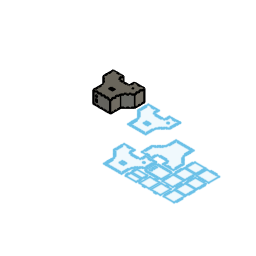
JD_BopIt_Enclosure (Autodesk Fusion 360 design; units mm, degrees)
Autodesk Fusion 360 part; units mm, degrees
(part 1 of 2)
sketch "Base" plane through (0, 0, 0) normal (0, 0, 1) x (1, 0, 0)
  line L0 (6.35, 14.5143) -> (6.35, 27.2143)
  line L1 (6.35, 27.2143) -> (0, 27.2143)
  line L2 (0, 39.9143) -> (6.35, 39.9143)
  line L3 (6.35, 39.9143) -> (6.35, 52.6143)
  line L4 (6.35, 52.6143) -> (0.1301, 52.6143)
  line L5 (0.1661, 65.1641) -> (0.1301, 52.6143)
  line L6 (0, 39.9143) -> (0, 27.2143)
  line L7 (6.35, 14.5143) -> (6.35, 27.2143)
  line L8 (6.35, 27.2143) -> (0, 27.2143)
  line L9 (31.7482, 0) -> (31.7482, 6.35)
  line L10 (31.7482, 6.35) -> (19.0482, 6.35)
  line L11 (19.0482, 6.35) -> (19.0482, 0)
  line L12 (57.1482, 6.35) -> (44.4482, 6.35)
  line L13 (44.4482, 6.35) -> (44.4482, 0)
  line L14 (57.1482, 0) -> (57.1482, 6.35)
  line L15 (82.5482, 6.35) -> (69.8482, 6.35)
  line L16 (69.8482, 6.35) -> (69.8482, 0)
  line L17 (82.5482, 0) -> (82.5482, 6.35)
  line L18 (107.9482, 6.35) -> (95.2482, 6.35)
  line L19 (95.2482, 6.35) -> (95.2482, 0)
  line L20 (107.9482, 0) -> (107.9482, 6.35)
  line L21 (31.7482, 0) -> (44.4482, 0)
  line L22 (57.1482, 0) -> (69.8482, 0)
  line L23 (82.5482, 0) -> (95.2482, 0)
  line L24 (107.9482, 0) -> (112.4857, 0)
  line L25 (6.35, 14.5143) -> (6.35, 27.2143)
  line L26 (6.35, 27.2143) -> (0, 27.2143)
  line L27 (0, 39.9143) -> (6.35, 39.9143)
  line L28 (6.35, 39.9143) -> (6.35, 52.6143)
  line L29 (6.35, 52.6143) -> (0, 52.6143)
  line L30 (6.35, 14.5143) -> (6.35, 27.2143)
  line L31 (6.35, 27.2143) -> (0, 27.2143)
  line L32 (0, 39.9143) -> (6.35, 39.9143)
  line L33 (6.35, 39.9143) -> (6.35, 52.6143)
  line L34 (6.35, 52.6143) -> (0, 52.6143)
  line L35 (127, 14.5143) -> (120.65, 14.5143)
  line L36 (120.65, 14.5143) -> (120.65, 27.2143)
  line L37 (120.65, 27.2143) -> (127, 27.2143)
  line L38 (127, 39.9143) -> (120.65, 39.9143)
  line L39 (120.65, 39.9143) -> (120.65, 52.6143)
  line L40 (120.65, 52.6143) -> (127, 52.6143)
  line L41 (127, 27.2143) -> (127, 39.9143)
  line L42 (127, 52.6143) -> (127, 65.0564)
  line L43 (19.0482, 0) -> (14.5107, 0)
  line L44 (6.35, 14.5143) -> (-0.0036, 14.5143)
  line L45 (152.6542, 98.2256) -> (148.1641, 93.7355)
  line L46 (148.1641, 93.7355) -> (143.6703, 98.2293)
  line L47 (143.6703, 98.2293) -> (134.69, 89.249)
  line L48 (134.69, 89.249) -> (139.1839, 84.7552)
  line L49 (157.1443, 102.7158) -> (152.6579, 107.2022)
  line L50 (152.6579, 107.2022) -> (161.6381, 116.1825)
  line L51 (161.6381, 116.1825) -> (166.1246, 111.696)
  line L52 (132.3139, 77.8854) -> (139.1838, 84.7552)
  line L53 (148.1641, 93.7355) -> (157.1443, 102.7158)
  line L54 (166.1246, 111.696) -> (173.0018, 118.5733)
  line L55 (178.3158, 148.5091) -> (171.9658, 148.5091)
  line L56 (171.9658, 148.5091) -> (171.9658, 135.8091)
  line L57 (171.9658, 135.8091) -> (178.3158, 135.8091)
  line L58 (178.3158, 154.8591) -> (178.3158, 161.2091)
  line L59 (178.3158, 161.2091) -> (171.9658, 161.2091)
  line L60 (171.9658, 161.2091) -> (171.9658, 173.9091)
  line L61 (171.9658, 173.9091) -> (178.3158, 173.9091)
  line L62 (178.3158, 131.4022) -> (178.3158, 135.8091)
  line L63 (178.3158, 148.5091) -> (178.3158, 161.2091)
  line L64 (178.3158, 173.9091) -> (178.3158, 178.3158)
  line L65 (146.3553, 196.4586) -> (146.3553, 190.1086)
  line L66 (146.3553, 190.1086) -> (133.6553, 190.1086)
  line L67 (133.6553, 190.1086) -> (133.6553, 196.4586)
  line L68 (160.1729, 196.4586) -> (146.3553, 196.4586)
  line L69 (133.6553, 196.4586) -> (119.8377, 196.4586)
  line L70 (82.855, 160.1729) -> (82.855, 153.8229)
  line L71 (82.855, 153.8229) -> (70.155, 153.8229)
  line L72 (70.155, 153.8229) -> (70.155, 160.1729)
  line L73 (82.855, 160.1729) -> (83.5515, 160.1729)
  line L74 (57.455, 153.8229) -> (57.455, 160.1729)
  line L75 (44.755, 153.8229) -> (57.455, 153.8229)
  line L76 (44.755, 160.1729) -> (44.755, 153.8229)
  line L77 (44.0586, 160.1729) -> (44.755, 160.1729)
  line L78 (57.455, 160.1729) -> (70.155, 160.1729)
  line L79 (-18.7452, 190.1086) -> (-6.0452, 190.1086)
  line L80 (-18.7452, 196.4634) -> (-18.7452, 190.1086)
  line L81 (-6.0452, 190.1086) -> (-6.0452, 196.4644)
  line L82 (7.766, 196.4654) -> (-6.0452, 196.4644)
  line L83 (-18.7452, 196.4634) -> (-32.1732, 196.4624)
  line L84 (-50.3446, 148.4522) -> (-43.9342, 148.4522)
  line L85 (-43.9342, 148.4522) -> (-43.9342, 135.7522)
  line L86 (-43.9342, 135.7522) -> (-50.3446, 135.7522)
  line L87 (-50.2805, 161.1522) -> (-43.9305, 161.1485)
  line L88 (-43.9305, 161.1485) -> (-43.9231, 173.8485)
  line L89 (-43.9231, 173.8485) -> (-50.2731, 173.8522)
  line L90 (-50.2731, 173.8522) -> (-50.3446, 173.8522)
  line L91 (-50.2805, 161.1522) -> (-50.3446, 161.1522)
  line L92 (-50.3446, 173.8522) -> (-50.3446, 178.3157)
  line L93 (-50.3446, 131.2946) -> (-50.3446, 135.7522)
  line L94 (-50.3446, 148.4522) -> (-50.3446, 161.1522)
  line L95 (-25.1571, 98.273) -> (-20.667, 93.7828)
  line L96 (-20.667, 93.7828) -> (-16.1768, 98.273)
  line L97 (-16.1768, 98.273) -> (-7.1966, 89.2927)
  line L98 (-7.1966, 89.2927) -> (-11.6867, 84.8026)
  line L99 (-25.1571, 107.2532) -> (-34.1373, 116.2335)
  line L100 (-34.1373, 116.2335) -> (-38.6275, 111.7433)
  line L101 (-29.6472, 102.7631) -> (-25.1571, 107.2532)
  line L102 (-45.3178, 118.4336) -> (-38.6275, 111.7433)
  line L103 (-29.6472, 102.7631) -> (-20.667, 93.7828)
  line L104 (-11.6867, 84.8026) -> (-4.9695, 78.0853)
  line L105 (25.9147, 171.9658) -> (25.9137, 160.1729)
  line L106 (25.9137, 160.1729) -> (44.0586, 160.1729)
  line L107 (101.6, 160.1729) -> (83.5515, 160.1729)
  line L108 (7.766, 196.4654) -> (25.9153, 196.4637)
  line L109 (25.9153, 196.4637) -> (25.9153, 184.6658)
  line L110 (119.8377, 196.4586) -> (101.7897, 196.5527)
  line L111 (101.7897, 196.5527) -> (101.7277, 184.6658)
  line L112 (-50.3446, 178.3157) -> (-50.346, 196.4624)
  line L113 (-50.346, 196.4624) -> (-32.1732, 196.4624)
  line L114 (160.1729, 196.4586) -> (178.3158, 196.4586)
  line L115 (178.3158, 196.4586) -> (178.3158, 196.4586)
  line L116 (178.3158, 196.4586) -> (160.1729, 196.4586)
  line L117 (160.1729, 196.4586) -> (160.1729, 196.4586)
  line L118 (178.3158, 178.3158) -> (178.3158, 178.3158)
  line L119 (178.3158, 178.3158) -> (178.3158, 196.4586)
  line L120 (178.3158, 196.4586) -> (178.3158, 196.4586)
  line L121 (178.3158, 196.4586) -> (178.3158, 178.3158)
  line L122 (-50.3446, 131.2946) -> (-50.3446, 123.4605)
  line L123 (-50.3446, 123.4605) -> (-45.3178, 118.4336)
  line L124 (-4.9695, 78.0853) -> (0.1661, 72.9498)
  line L125 (0.1661, 72.9498) -> (0.1661, 65.1641)
  line L126 (178.3158, 131.4022) -> (178.3158, 123.8872)
  line L127 (178.3158, 123.8872) -> (173.0018, 118.5733)
  line L128 (132.3139, 77.8854) -> (127, 72.5714)
  line L129 (127, 72.5714) -> (127, 65.0564)
  line L130 (-0.0036, 14.5143) -> (0, 0)
  line L131 (0, 0) -> (14.5107, 0)
  line L132 (112.4857, 0) -> (127, 0)
  line L133 (127, 0) -> (127, 14.5143)
  line L134 (25.9153, 184.6658) -> (19.5653, 184.6658)
  line L135 (19.5653, 184.6658) -> (19.5653, 171.9658)
  line L136 (19.5653, 171.9658) -> (25.9153, 171.9658)
  line L137 (101.6948, 184.6658) -> (108.0448, 184.6658)
  line L138 (108.0448, 184.6658) -> (108.0448, 171.9658)
  line L139 (108.0448, 171.9658) -> (101.6948, 171.9658)
  line L140 (101.6, 160.1729) -> (101.6948, 171.9658)
  dimension "d43" = 6.35
  dimension "d44" = 12.7
  constraint vertical L93
  constraint coincident L51.end L52
  constraint collinear L68 L69
  constraint collinear L73 L77
  constraint collinear L77 L78
  constraint collinear L82 L83
  constraint horizontal L84
  constraint vertical L85
  constraint horizontal L86
  constraint coincident L90.end L93
  constraint perpendicular L90 L93
  constraint perpendicular L91 L93
  constraint collinear L92 L93
  constraint collinear L93 L94
  constraint parallel L95 L102
  constraint perpendicular L95 L96
  constraint perpendicular L96 L97
  constraint coincident L98.end L102
  constraint perpendicular L98 L102
  constraint collinear L102 L103
  constraint collinear L103 L104
  constraint horizontal L106
  constraint horizontal L107
  constraint perpendicular L105 L108
  constraint vertical L109
  constraint perpendicular L83 L112
  constraint horizontal L113
  constraint horizontal L114
  constraint horizontal L116
  constraint vertical L119
  constraint vertical L121
  constraint perpendicular L86 L122
  constraint parallel L102 L123
  constraint parallel L104 L124
  constraint vertical L125
  constraint parallel L62 L126
  constraint parallel L54 L127
  constraint parallel L52 L128
  constraint parallel L42 L129
  constraint coincident L130.end L131.start
  constraint parallel L43 L131
  constraint parallel L35 L132
  constraint perpendicular L35 L133
  constraint horizontal L134
  constraint vertical L135
  constraint horizontal L136
  constraint coincident L136 L105.start
  constraint coincident L137 L111.end
  measures "d43" distance of L95.end L96.end
  measures "d44" distance of L96.end L97.end
extrude "Extrude1" add sketch "Base" along normal blind 6.35 makes body 1
sketch "Walls" plane through (0, 0, 0) normal (0, 0, 1) x (1, 0, 0)
  line L0 (137.6256, 467.2914) -> (137.6256, 473.6471)
  line L1 (67.9035, 520.7146) -> (61.4925, 520.7146)
  line L2 (124.9256, 467.2914) -> (137.6256, 467.2914)
  line L3 (67.9147, 558.8109) -> (61.5647, 558.8146)
  line L4 (67.9035, 533.4146) -> (67.9035, 520.7146)
  line L5 (61.4925, 516.257) -> (61.4925, 508.4229)
  line L6 (61.4925, 533.4146) -> (61.4925, 546.1146)
  line L7 (61.5647, 558.8146) -> (61.4925, 558.8146)
  line L8 (61.4925, 516.257) -> (61.4925, 520.7146)
  line L9 (124.9256, 473.6462) -> (124.9256, 467.2914)
  line L10 (67.9073, 546.1109) -> (67.9147, 558.8109)
  line L11 (61.4925, 533.4146) -> (67.9035, 533.4146)
  line L12 (61.5573, 546.1146) -> (67.9073, 546.1109)
  line L13 (61.5573, 546.1146) -> (61.4925, 546.1146)
  line L14 (163.2361, 473.6452) -> (163.2361, 549.8452)
  line L15 (93.3255, 549.8452) -> (93.3255, 473.6452)
  line L16 (93.3255, 473.6452) -> (124.9256, 473.6452)
  line L17 (137.6256, 473.6452) -> (163.2361, 473.6452)
  line L18 (61.5647, 558.8146) -> (61.4925, 558.8146)
  line L19 (61.4925, 546.1146) -> (61.5573, 546.1146)
  line L20 (166.3289, 377.2551) -> (90.1289, 377.2551)
  line L21 (90.1289, 377.2551) -> (90.1289, 389.0479)
  line L22 (83.7789, 389.0479) -> (90.1289, 389.0479)
  line L23 (83.7789, 401.7479) -> (83.7789, 389.0479)
  line L24 (90.1289, 401.7479) -> (83.7789, 401.7479)
  line L25 (90.1289, 413.5459) -> (166.3289, 413.5459)
  line L26 (90.1289, 413.5459) -> (90.1289, 401.7479)
  line L27 (172.9027, 434.1418) -> (172.9027, 446.8418)
  line L28 (172.9027, 446.8418) -> (166.5527, 446.8418)
  line L29 (90.3527, 458.6347) -> (166.5527, 458.6347)
  line L30 (166.5527, 422.3438) -> (90.3527, 422.3438)
  line L31 (166.5527, 458.6347) -> (166.5527, 446.8418)
  line L32 (166.5527, 434.1418) -> (172.9027, 434.1418)
  line L33 (166.5527, 422.3438) -> (166.5527, 434.1418)
  line L34 (61.4925, 572.3515) -> (61.5647, 558.8146)
  line L35 (241.065, 580.6993) -> (241.065, 656.8993)
  line L36 (171.1543, 580.6993) -> (202.7545, 580.6993)
  line L37 (202.7545, 574.3454) -> (215.4545, 574.3454)
  line L38 (215.4545, 580.6993) -> (241.065, 580.6993)
  line L39 (171.1543, 656.8993) -> (171.1543, 580.6993)
  line L40 (215.4545, 574.3454) -> (215.4545, 580.7012)
  line L41 (202.7545, 580.7002) -> (202.7545, 574.3454)
  line L42 (160.9039, 571.0581) -> (160.9039, 647.2581)
  line L43 (72.357, 647.2581) -> (72.357, 571.0581)
  line L44 (97.6142, 564.7081) -> (110.3142, 564.7081)
  line L45 (110.3142, 564.7081) -> (110.3142, 571.0581)
  line L46 (97.6142, 571.0581) -> (97.6142, 564.7081)
  line L47 (135.7142, 571.0581) -> (135.7142, 564.7081)
  line L48 (123.0142, 564.7081) -> (123.0142, 571.0581)
  line L49 (135.7142, 564.7081) -> (123.0142, 564.7081)
  line L50 (72.357, 571.0581) -> (97.6142, 571.0581)
  line L51 (110.3142, 571.0581) -> (123.0142, 571.0581)
  line L52 (135.7142, 571.0581) -> (160.9039, 571.0581)
  line L53 (225.2765, 415.9992) -> (301.4765, 415.9992)
  line L54 (301.4765, 337.0777) -> (225.2765, 337.0777)
  line L55 (218.9265, 389.692) -> (225.2765, 389.692)
  line L56 (218.9265, 351.592) -> (218.9265, 364.292)
  line L57 (218.9265, 364.292) -> (225.2765, 364.292)
  line L58 (225.2765, 351.592) -> (218.9265, 351.592)
  line L59 (225.2765, 376.992) -> (218.9265, 376.992)
  line L60 (218.9265, 376.992) -> (218.9265, 389.692)
  line L61 (225.2765, 389.692) -> (225.2765, 415.9992)
  line L62 (225.2765, 337.0777) -> (225.2765, 351.592)
  line L63 (225.2765, 364.292) -> (225.2765, 376.992)
  line L64 (300.954, 497.2393) -> (224.754, 497.2393)
  line L65 (224.754, 424.6679) -> (300.954, 424.6679)
  line L66 (224.754, 432.1829) -> (224.754, 441.8984)
  line L67 (224.754, 454.5984) -> (224.754, 467.2984)
  line L68 (224.754, 460.9484) -> (224.754, 454.5984)
  line L69 (224.754, 432.1829) -> (224.754, 424.6679)
  line L70 (218.3988, 441.8984) -> (224.7541, 441.8984)
  line L71 (218.3988, 454.5984) -> (218.3988, 441.8984)
  line L72 (224.754, 454.5984) -> (218.3988, 454.5984)
  line L73 (224.754, 467.2984) -> (218.4092, 467.2984)
  line L74 (224.754, 479.9984) -> (224.754, 489.7243)
  line L75 (218.4092, 467.2984) -> (218.4092, 479.9984)
  line L76 (224.754, 497.2393) -> (224.754, 489.7243)
  line L77 (218.4092, 479.9984) -> (224.754, 479.9984)
  line L78 (-12.5432, 340.4938) -> (63.6568, 340.4938)
  line L79 (63.6568, 355.0081) -> (70.0068, 355.0081)
  line L80 (70.0068, 380.4081) -> (70.0068, 393.1081)
  line L81 (63.6568, 393.1081) -> (63.6568, 419.4152)
  line L82 (70.0068, 367.7081) -> (63.6568, 367.7081)
  line L83 (70.0068, 393.1081) -> (63.6568, 393.1081)
  line L84 (70.0068, 355.0081) -> (70.0068, 367.7081)
  line L85 (63.6568, 380.4081) -> (70.0068, 380.4081)
  line L86 (63.6568, 419.4152) -> (-12.5432, 419.4152)
  line L87 (63.6568, 340.4938) -> (63.6568, 355.0081)
  line L88 (63.6568, 367.7081) -> (63.6568, 380.4081)
  line L89 (61.5367, 434.5839) -> (61.5367, 427.0688)
  line L90 (61.5367, 456.9994) -> (61.5367, 469.6994)
  line L91 (61.5367, 463.3494) -> (61.5367, 456.9994)
  line L92 (67.8919, 456.9994) -> (67.8919, 444.2994)
  line L93 (61.5367, 482.3994) -> (61.5367, 492.1253)
  line L94 (61.5367, 456.9994) -> (67.8919, 456.9994)
  line L95 (61.5367, 499.6403) -> (61.5367, 492.1253)
  line L96 (67.8815, 469.6994) -> (67.8815, 482.3994)
  line L97 (-14.6633, 499.6403) -> (61.5367, 499.6403)
  line L98 (67.8919, 444.2994) -> (61.5366, 444.2994)
  line L99 (61.5367, 434.5839) -> (61.5367, 444.2994)
  line L100 (61.5367, 427.0688) -> (-14.6633, 427.0688)
  line L101 (67.8815, 482.3994) -> (61.5367, 482.3994)
  line L102 (61.5367, 469.6994) -> (67.8815, 469.6994)
  line L103 (199.4678, 353.0616) -> (199.4678, 276.8616)
  line L104 (85.1678, 276.8616) -> (85.1678, 353.0616)
  line L105 (174.066, 359.41) -> (174.066, 353.06)
  line L106 (110.566, 359.41) -> (97.866, 359.41)
  line L107 (161.366, 353.06) -> (174.066, 353.06)
  line L108 (148.666, 359.41) -> (148.666, 353.06)
  line L109 (186.766, 359.41) -> (174.066, 359.41)
  line L110 (110.566, 353.06) -> (110.566, 359.41)
  line L111 (161.366, 353.06) -> (161.366, 359.41)
  line L112 (135.966, 353.06) -> (135.966, 359.41)
  line L113 (97.866, 359.41) -> (97.866, 353.06)
  line L114 (186.766, 353.06) -> (186.766, 359.41)
  line L115 (123.266, 359.41) -> (123.266, 353.06)
  line L116 (135.966, 353.06) -> (148.666, 353.06)
  line L117 (161.366, 359.41) -> (148.666, 359.41)
  line L118 (135.966, 359.41) -> (123.266, 359.41)
  line L119 (110.566, 353.06) -> (123.266, 353.06)
  line L120 (85.1678, 353.0616) -> (97.866, 353.06)
  line L121 (186.766, 353.06) -> (199.4678, 353.0616)
  line L122 (-12.5432, 355.0081) -> (-18.8932, 355.0081)
  line L123 (-12.5432, 380.4081) -> (-18.8932, 380.4081)
  line L124 (-18.8932, 355.0081) -> (-18.8932, 367.7081)
  line L125 (-18.8932, 380.4081) -> (-18.8932, 393.1081)
  line L126 (-18.8932, 393.1081) -> (-12.5432, 393.1081)
  line L127 (-18.8932, 367.7081) -> (-12.5432, 367.7081)
  line L128 (-21.0185, 444.2994) -> (-14.6632, 444.2994)
  line L129 (-14.6633, 469.6994) -> (-21.0081, 469.6994)
  line L130 (-21.0081, 469.6994) -> (-21.0081, 482.3994)
  line L131 (-14.6633, 456.9994) -> (-21.0185, 456.9994)
  line L132 (-21.0185, 456.9994) -> (-21.0185, 444.2994)
  line L133 (-21.0081, 482.3994) -> (-14.6633, 482.3994)
  line L134 (-21.1186, 533.4146) -> (-21.1186, 520.7146)
  line L135 (-14.7075, 533.4146) -> (-21.1186, 533.4146)
  line L136 (-21.1186, 520.7146) -> (-14.7075, 520.7146)
  line L137 (-14.7723, 546.1146) -> (-21.1223, 546.1109)
  line L138 (-21.1223, 546.1109) -> (-21.1298, 558.8109)
  line L139 (-21.1298, 558.8109) -> (-14.7798, 558.8146)
  line L140 (-14.7075, 520.7146) -> (-14.7075, 508.4229)
  line L141 (-14.6633, 482.3994) -> (-14.6633, 499.6403)
  line L142 (-14.6633, 427.0688) -> (-14.6633, 444.2994)
  line L143 (-14.6633, 456.9994) -> (-14.6633, 469.6994)
  line L144 (-12.5432, 355.0081) -> (-12.5432, 340.4938)
  line L145 (-12.5432, 419.4152) -> (-12.5432, 393.1081)
  line L146 (-12.5432, 380.4081) -> (-12.5432, 367.7081)
  line L147 (61.4925, 572.3515) -> (-14.7798, 571.9445)
  line L148 (-14.7798, 571.9445) -> (-14.7798, 558.8146)
  line L149 (-14.7723, 546.1146) -> (-14.7075, 533.4146)
  line L150 (186.766, 276.8632) -> (186.766, 270.5132)
  line L151 (123.266, 270.5132) -> (123.266, 276.8632)
  line L152 (161.366, 270.5132) -> (148.666, 270.5132)
  line L153 (110.566, 270.5132) -> (97.866, 270.5132)
  line L154 (135.966, 276.8632) -> (135.966, 270.5132)
  line L155 (135.966, 270.5132) -> (123.266, 270.5132)
  line L156 (174.066, 270.5132) -> (174.066, 276.8632)
  line L157 (186.766, 270.5132) -> (174.066, 270.5132)
  line L158 (161.366, 276.8632) -> (161.366, 270.5132)
  line L159 (148.666, 270.5132) -> (148.666, 276.8632)
  line L160 (110.566, 276.8632) -> (110.566, 270.5132)
  line L161 (97.866, 270.5132) -> (97.866, 276.8632)
  line L162 (97.866, 276.8616) -> (85.1678, 276.8616)
  line L163 (123.266, 276.8616) -> (110.566, 276.8616)
  line L164 (148.666, 276.8616) -> (135.966, 276.8616)
  line L165 (199.4678, 276.8616) -> (186.766, 276.8616)
  line L166 (174.066, 276.8616) -> (161.366, 276.8616)
  line L167 (307.8265, 376.992) -> (307.8265, 389.692)
  line L168 (307.8265, 389.692) -> (301.4765, 389.692)
  line L169 (301.4765, 351.592) -> (307.8265, 351.592)
  line L170 (307.8265, 364.292) -> (301.4765, 364.292)
  line L171 (307.8265, 351.592) -> (307.8265, 364.292)
  line L172 (301.4765, 376.992) -> (307.8265, 376.992)
  line L173 (301.4765, 351.592) -> (301.4765, 337.0777)
  line L174 (301.4765, 415.9992) -> (301.4765, 389.692)
  line L175 (301.4765, 376.992) -> (301.4765, 364.292)
  line L176 (307.3092, 454.5984) -> (307.3092, 441.8984)
  line L177 (300.954, 467.2984) -> (307.2988, 467.2984)
  line L178 (307.2988, 479.9984) -> (300.954, 479.9984)
  line L179 (300.954, 454.5984) -> (307.3092, 454.5984)
  line L180 (307.2988, 467.2984) -> (307.2988, 479.9984)
  line L181 (307.3092, 441.8984) -> (300.9538, 441.8984)
  line L182 (300.954, 479.9984) -> (300.954, 497.2393)
  line L183 (300.954, 424.6679) -> (300.954, 441.8984)
  line L184 (300.954, 454.5984) -> (300.954, 467.2984)
  line L185 (124.9256, 556.1991) -> (137.6256, 556.1991)
  line L186 (137.6256, 556.1991) -> (137.6256, 549.8433)
  line L187 (124.9256, 549.8442) -> (124.9256, 556.1991)
  line L188 (202.7545, 656.8983) -> (202.7545, 663.2531)
  line L189 (215.4545, 663.2531) -> (215.4545, 656.8973)
  line L190 (202.7545, 663.2531) -> (215.4545, 663.2531)
  line L191 (135.7142, 647.2581) -> (135.7142, 653.608)
  line L192 (110.3142, 653.608) -> (110.3142, 647.2581)
  line L193 (97.6142, 647.2581) -> (97.6142, 653.608)
  line L194 (135.7142, 653.608) -> (123.0142, 653.608)
  line L195 (123.0142, 653.608) -> (123.0142, 647.2581)
  line L196 (97.6142, 653.608) -> (110.3142, 653.608)
  line L197 (163.2361, 549.8452) -> (137.6256, 549.8452)
  line L198 (124.9256, 549.8452) -> (93.3255, 549.8452)
  line L199 (97.6142, 647.2581) -> (72.357, 647.2581)
  line L200 (160.9039, 647.2581) -> (135.7142, 647.2581)
  line L201 (123.0142, 647.2581) -> (110.3142, 647.2581)
  line L202 (241.065, 656.8993) -> (215.4545, 656.8993)
  line L203 (202.7545, 656.8993) -> (171.1543, 656.8993)
  line L204 (172.6789, 401.7479) -> (172.6789, 389.0479)
  line L205 (166.3289, 401.7479) -> (172.6789, 401.7479)
  line L206 (172.6789, 389.0479) -> (166.3289, 389.0479)
  line L207 (90.3527, 434.1418) -> (84.0027, 434.1418)
  line L208 (84.0027, 446.8418) -> (90.3527, 446.8418)
  line L209 (84.0027, 434.1418) -> (84.0027, 446.8418)
  line L210 (166.3289, 413.5459) -> (166.3289, 401.7479)
  line L211 (166.3289, 389.0479) -> (166.3289, 377.2551)
  line L212 (90.3527, 422.3438) -> (90.3527, 434.1418)
  line L213 (90.3527, 446.8418) -> (90.3527, 458.6347)
  line L214 (-14.7075, 508.4229) -> (-14.7075, 504.4605)
  line L215 (-14.7075, 504.4605) -> (61.4925, 504.4605)
  line L216 (61.4925, 504.4605) -> (61.4925, 508.4229)
  line L217 (226.5277, 546.1146) -> (226.5925, 533.4146)
  line L218 (220.1814, 520.7146) -> (226.5925, 520.7146)
  line L219 (302.7925, 504.4605) -> (302.7925, 508.4229)
  line L220 (302.7925, 572.3515) -> (302.8647, 558.8146)
  line L221 (302.7925, 546.1146) -> (302.8573, 546.1146)
  line L222 (226.5277, 546.1146) -> (220.1777, 546.1109)
  line L223 (302.7925, 533.4146) -> (302.7925, 546.1146)
  line L224 (220.1814, 533.4146) -> (220.1814, 520.7146)
  line L225 (302.7925, 516.257) -> (302.7925, 508.4229)
  line L226 (302.8647, 558.8146) -> (302.7925, 558.8146)
  line L227 (302.7925, 533.4146) -> (309.2035, 533.4146)
  line L228 (302.8573, 546.1146) -> (302.7925, 546.1146)
  line L229 (309.2035, 520.7146) -> (302.7925, 520.7146)
  line L230 (220.1702, 558.8109) -> (226.5202, 558.8146)
  line L231 (302.7925, 516.257) -> (302.7925, 520.7146)
  line L232 (226.5202, 571.9445) -> (226.5202, 558.8146)
  line L233 (302.7925, 572.3515) -> (226.5202, 571.9445)
  line L234 (226.5925, 508.4229) -> (226.5925, 504.4605)
  line L235 (309.2147, 558.8109) -> (302.8647, 558.8146)
  line L236 (226.5925, 533.4146) -> (220.1814, 533.4146)
  line L237 (302.8647, 558.8146) -> (302.7925, 558.8146)
  line L238 (220.1777, 546.1109) -> (220.1702, 558.8109)
  line L239 (226.5925, 520.7146) -> (226.5925, 508.4229)
  line L240 (302.8573, 546.1146) -> (309.2073, 546.1109)
  line L241 (309.2035, 533.4146) -> (309.2035, 520.7146)
  line L242 (309.2073, 546.1109) -> (309.2147, 558.8109)
  line L243 (226.5925, 504.4605) -> (302.7925, 504.4605)
  line L244 (109.7658, 336.7323) -> (97.9658, 336.7323)
  line L245 (97.9658, 336.7323) -> (97.9658, 316.6323)
  line L246 (97.9658, 316.6323) -> (109.7658, 316.6323)
  line L247 (109.7658, 316.6323) -> (109.7658, 336.7323)
  circle A0 centre (103.4158, 298.7439) radius 7.75
  point P0 (78.8178, 353.06)
  dimension "d55" = 76.2
  dimension "d59" = 76.2
  dimension "d61" = 76.2
  dimension "d62" = 76.2
  dimension "d63" = 76.2
  dimension "d66" = 76.2
  dimension "d68" = 76.2
  dimension "d73" = 76.2
  dimension "d141" = 3.9624
  dimension "d143" = 3.9624
  dimension "d152" = 11.8
  dimension "d153" = 20.1
  dimension "d154" = 15.5
  constraint vertical L8
  constraint horizontal L11
  constraint vertical L4
  constraint horizontal L1
  constraint coincident L7.end L8
  constraint perpendicular L7 L8
  constraint perpendicular L8 L13
  constraint collinear L6 L8
  constraint perpendicular L1 L5
  constraint horizontal L16
  constraint vertical L14
  constraint horizontal L197
  constraint vertical L15
  constraint coincident L9 L16.end
  constraint coincident L0 L17.start
  constraint collinear L16 L17
  constraint vertical L26
  constraint horizontal L24
  constraint vertical L23
  constraint horizontal L22
  constraint horizontal L25
  constraint vertical L210
  constraint horizontal L20
  constraint vertical L21
  constraint horizontal L36
  constraint vertical L35
  constraint horizontal L202
  constraint vertical L39
  constraint coincident L36.end L41
  constraint coincident L38.start L40
  constraint collinear L36 L38
  constraint horizontal L50
  constraint vertical L42
  constraint horizontal L200
  constraint vertical L43
  constraint collinear L50 L51
  constraint coincident L47 L52.start
  constraint collinear L51 L52
  constraint horizontal L53
  constraint vertical L174
  constraint horizontal L54
  constraint vertical L62
  constraint collinear L61 L62
  constraint collinear L62 L63
  constraint coincident L74.start L66
  constraint parallel L74 L76
  constraint parallel L66 L69
  constraint perpendicular L65 L69
  constraint perpendicular L65 L183
  constraint perpendicular L64 L76
  constraint symmetric L87.start L78 L78.end
  constraint symmetric L144.end L78 L78.start
  constraint vertical L103
  constraint horizontal L165
  constraint vertical L104
  constraint collinear L141 L142
  constraint coincident L128 L142.end
  constraint collinear L142 L143
  constraint collinear L144 L145
  constraint collinear L145 L146
  constraint perpendicular L34 L147
  constraint vertical L148
  constraint coincident L160 L163.end
  constraint coincident L161 L162.start
  constraint collinear L162 L165
  constraint coincident L154 L164.end
  constraint coincident L151 L163.start
  constraint collinear L163 L165
  constraint coincident L158 L166.end
  constraint coincident L159 L164.start
  constraint collinear L164 L165
  constraint coincident L150 L165.end
  constraint coincident L156 L166.start
  constraint collinear L165 L166
  constraint collinear L173 L174
  constraint collinear L174 L175
  constraint collinear L182 L183
  constraint coincident L181 L183.end
  constraint collinear L183 L184
  constraint coincident L186 L197.end
  constraint coincident L187 L198.start
  constraint collinear L197 L198
  constraint collinear L199 L200
  constraint collinear L200 L201
  constraint coincident L189 L202.end
  constraint coincident L188 L203.start
  constraint collinear L202 L203
  constraint collinear L210 L211
  constraint collinear L212 L213
  constraint parallel L140 L214
  constraint perpendicular L5 L215
  constraint perpendicular L215 L216
  constraint vertical L231
  constraint horizontal L227
  constraint vertical L241
  constraint horizontal L229
  constraint coincident L226.end L231
  constraint perpendicular L231 L237
  constraint perpendicular L228 L231
  constraint collinear L223 L231
  constraint perpendicular L225 L229
  constraint perpendicular L220 L233
  constraint vertical L232
  constraint parallel L234 L239
  constraint perpendicular L225 L243
  constraint perpendicular L219 L243
  measures "d55" distance of L15.end L15.start
  measures "d59" distance of L25.end L25.start
  measures "d61" distance of L30.end L30.start
  measures "d62" distance of L39.start L36.start
  measures "d63" distance of L43.end L43.start
  measures "d66" distance of L53.start L53.end
  measures "d68" distance of L65.end L65.start
  measures "d73" distance of L104.end L104.start
  measures "d141" distance of L140.end L214.end
  measures "d143" distance of L234.start L234.end
  measures "d152" distance of L244.start L244.end
  measures "d153" distance of L244.start L246.end
  measures "d154" diameter of A0
sketch "Top" plane through (0, 0, 0) normal (0, 0, 1) x (1, 0, 0)
  line L0 (210.0658, 148.4522) -> (210.0658, 135.7522)
  line L1 (381, 72.5714) -> (381, 65.0564)
  line L2 (261.766, 196.4654) -> (279.9153, 196.4637)
  line L3 (373.8377, 196.4516) -> (355.7896, 196.546)
  line L4 (254.1661, 72.9498) -> (254.1661, 65.1641)
  line L5 (254, 39.9143) -> (260.35, 39.9143)
  line L6 (402.1641, 93.7355) -> (397.6703, 98.2293)
  line L7 (210.0658, 135.7522) -> (203.6554, 135.7522)
  line L8 (425.9658, 148.5091) -> (425.9658, 135.8091)
  line L9 (203.6554, 148.4522) -> (203.6554, 161.1522)
  line L10 (203.6554, 123.4605) -> (208.6822, 118.4336)
  line L11 (355.6948, 184.6658) -> (362.0448, 184.6658)
  line L12 (228.8429, 107.2532) -> (219.8627, 116.2335)
  line L13 (260.35, 52.6143) -> (254, 52.6143)
  line L14 (249.0305, 78.0853) -> (254.1661, 72.9498)
  line L15 (224.3528, 102.7631) -> (228.8429, 107.2532)
  line L16 (311.1482, 6.35) -> (298.4482, 6.35)
  line L17 (210.0695, 161.1485) -> (210.0769, 173.8485)
  line L18 (273.5653, 171.9658) -> (279.9153, 171.9658)
  line L19 (233.333, 93.7828) -> (237.8232, 98.273)
  line L20 (355.6, 160.1729) -> (337.5515, 160.1729)
  line L21 (235.2548, 190.1086) -> (247.9548, 190.1086)
  line L22 (208.6822, 118.4336) -> (215.3725, 111.7433)
  line L23 (432.1088, 196.4461) -> (413.7585, 196.4461)
  line L24 (210.0769, 173.8485) -> (203.7269, 173.8522)
  line L25 (203.6554, 148.4522) -> (210.0658, 148.4522)
  line L26 (203.6554, 131.2946) -> (203.6554, 123.4605)
  line L27 (219.8627, 116.2335) -> (215.3725, 111.7433)
  line L28 (246.8034, 89.2927) -> (242.3133, 84.8026)
  line L29 (235.2548, 196.4634) -> (235.2548, 190.1086)
  line L30 (260.35, 52.6143) -> (254, 52.6143)
  line L31 (228.8429, 98.273) -> (233.333, 93.7828)
  line L32 (254, 39.9143) -> (260.35, 39.9143)
  line L33 (247.9548, 190.1086) -> (247.9548, 196.4644)
  line L34 (203.6554, 131.2946) -> (203.6554, 135.7522)
  line L35 (406.6579, 107.2022) -> (415.6381, 116.1825)
  line L36 (203.6554, 178.3157) -> (203.654, 196.4624)
  line L37 (203.6554, 173.8522) -> (203.6554, 178.3157)
  line L38 (387.6553, 190.1086) -> (387.6553, 196.4513)
  line L39 (237.8232, 98.273) -> (246.8034, 89.2927)
  line L40 (298.755, 160.1729) -> (298.755, 153.8229)
  line L41 (336.5482, 6.35) -> (323.8482, 6.35)
  line L42 (260.35, 39.9143) -> (260.35, 52.6143)
  line L43 (387.6553, 196.4513) -> (373.8377, 196.4516)
  line L44 (355.6, 160.1729) -> (355.6948, 171.9658)
  line L45 (413.7643, 196.4509) -> (432.1145, 196.4509)
  line L46 (432.3158, 148.5091) -> (425.9658, 148.5091)
  line L47 (402.1641, 93.7355) -> (411.1443, 102.7158)
  line L48 (397.6703, 98.2293) -> (388.69, 89.249)
  line L49 (425.9658, 161.2091) -> (425.9658, 173.9091)
  line L50 (311.1482, 0) -> (311.1482, 6.35)
  line L51 (361.9482, 0) -> (361.9482, 6.35)
  line L52 (279.9137, 160.1729) -> (298.0586, 160.1729)
  line L53 (432.3158, 154.8591) -> (432.3158, 161.2091)
  line L54 (260.35, 39.9143) -> (260.35, 52.6143)
  line L55 (432.3158, 131.4022) -> (432.3158, 123.8872)
  line L56 (336.855, 160.1729) -> (337.5515, 160.1729)
  line L57 (432.3158, 148.5091) -> (432.3158, 161.2091)
  line L58 (254, 0) -> (268.5107, 0)
  line L59 (273.0482, 6.35) -> (273.0482, 0)
  line L60 (381, 27.2143) -> (381, 39.9143)
  line L61 (260.35, 27.2143) -> (254, 27.2143)
  line L62 (425.9658, 173.9091) -> (432.3158, 173.9091)
  line L63 (336.855, 153.8229) -> (324.155, 153.8229)
  line L64 (374.65, 14.5143) -> (374.65, 27.2143)
  line L65 (432.3158, 161.2091) -> (425.9658, 161.2091)
  line L66 (420.1246, 111.696) -> (427.0018, 118.5733)
  line L67 (311.455, 153.8229) -> (311.455, 160.1729)
  line L68 (361.9482, 0) -> (366.4857, 0)
  line L69 (432.1145, 196.4509) -> (432.1088, 196.4461)
  line L70 (336.855, 160.1729) -> (336.855, 153.8229)
  line L71 (432.3158, 178.3158) -> (432.1088, 178.3158)
  line L72 (260.35, 27.2143) -> (254, 27.2143)
  line L73 (432.3158, 131.4022) -> (432.3158, 135.8091)
  line L74 (432.1088, 178.3158) -> (432.1088, 196.4461)
  line L75 (260.35, 14.5143) -> (260.35, 27.2143)
  line L76 (298.0586, 160.1729) -> (298.755, 160.1729)
  line L77 (411.1443, 102.7158) -> (406.6579, 107.2022)
  line L78 (381, 14.5143) -> (374.65, 14.5143)
  line L79 (362.0448, 184.6658) -> (362.0448, 171.9658)
  line L80 (432.1088, 196.4461) -> (432.3158, 196.4461)
  line L81 (381, 0) -> (381, 14.5143)
  line L82 (432.3158, 196.4461) -> (432.3158, 178.3158)
  line L83 (366.4857, 0) -> (381, 0)
  line L84 (381, 52.6143) -> (381, 65.0564)
  line L85 (311.455, 160.1729) -> (324.155, 160.1729)
  line L86 (406.6542, 98.2256) -> (402.1641, 93.7355)
  line L87 (381, 39.9143) -> (374.65, 39.9143)
  line L88 (374.65, 27.2143) -> (381, 27.2143)
  line L89 (374.65, 39.9143) -> (374.65, 52.6143)
  line L90 (432.3158, 173.9091) -> (432.3158, 178.3158)
  line L91 (260.35, 14.5143) -> (260.35, 27.2143)
  line L92 (374.65, 52.6143) -> (381, 52.6143)
  line L93 (324.155, 153.8229) -> (324.155, 160.1729)
  line L94 (285.7482, 0) -> (298.4482, 0)
  line L95 (279.9153, 184.6658) -> (273.5653, 184.6658)
  line L96 (260.35, 14.5143) -> (253.9964, 14.5143)
  line L97 (388.69, 89.249) -> (393.1839, 84.7552)
  line L98 (386.3139, 77.8854) -> (393.1838, 84.7552)
  line L99 (273.0482, 0) -> (268.5107, 0)
  line L100 (260.35, 14.5143) -> (260.35, 27.2143)
  line L101 (415.6381, 116.1825) -> (420.1246, 111.696)
  line L102 (298.4482, 6.35) -> (298.4482, 0)
  line L103 (260.35, 14.5143) -> (260.35, 27.2143)
  line L104 (203.7195, 161.1522) -> (203.6554, 161.1522)
  line L105 (273.5653, 184.6658) -> (273.5653, 171.9658)
  line L106 (298.755, 153.8229) -> (311.455, 153.8229)
  line L107 (203.7195, 161.1522) -> (210.0695, 161.1485)
  line L108 (203.654, 196.4624) -> (221.8268, 196.4624)
  line L109 (311.1482, 0) -> (323.8482, 0)
  line L110 (260.35, 39.9143) -> (260.35, 52.6143)
  line L111 (242.3133, 84.8026) -> (249.0305, 78.0853)
  line L112 (413.7643, 196.4509) -> (400.3553, 196.4511)
  line L113 (336.5482, 0) -> (349.2482, 0)
  line L114 (235.2548, 196.4634) -> (221.8268, 196.4624)
  line L115 (261.766, 196.4654) -> (247.9548, 196.4644)
  line L116 (400.3553, 190.1086) -> (387.6553, 190.1086)
  line L117 (224.3528, 102.7631) -> (233.333, 93.7828)
  line L118 (254.1661, 65.1641) -> (254.1301, 52.6143)
  line L119 (203.7269, 173.8522) -> (203.6554, 173.8522)
  line L120 (323.8482, 6.35) -> (323.8482, 0)
  line L121 (413.7585, 196.4461) -> (413.7643, 196.4509)
  line L122 (355.7896, 196.546) -> (355.7277, 184.6658)
  line L123 (386.3139, 77.8854) -> (381, 72.5714)
  line L124 (400.3553, 196.4511) -> (400.3553, 190.1086)
  line L125 (254, 39.9143) -> (254, 27.2143)
  line L126 (349.2482, 6.35) -> (349.2482, 0)
  line L127 (254, 39.9143) -> (260.35, 39.9143)
  line L128 (260.35, 52.6143) -> (254.1301, 52.6143)
  line L129 (336.5482, 0) -> (336.5482, 6.35)
  line L130 (361.9482, 6.35) -> (349.2482, 6.35)
  line L131 (279.9153, 196.4637) -> (279.9153, 184.6658)
  line L132 (279.9147, 171.9658) -> (279.9137, 160.1729)
  line L133 (362.0448, 171.9658) -> (355.6948, 171.9658)
  line L134 (260.35, 27.2143) -> (254, 27.2143)
  line L135 (253.9964, 14.5143) -> (254, 0)
  line L136 (432.3158, 123.8872) -> (427.0018, 118.5733)
  line L137 (425.9658, 135.8091) -> (432.3158, 135.8091)
  line L138 (285.7482, 0) -> (285.7482, 6.35)
  line L139 (285.7482, 6.35) -> (273.0482, 6.35)
  line L140 (260.35, 27.2143) -> (254, 27.2143)
  circle A0 centre (390.6105, 151.4522) radius 4.83
  line L141 (303.8592, 63.4148) -> (316.4292, 63.4148)
  line L142 (316.4292, 63.4148) -> (316.4292, 82.4848)
  line L143 (316.4292, 82.4848) -> (303.8592, 82.4848)
  line L144 (303.8592, 82.4848) -> (303.8592, 63.4148)
  line L145 (331.6692, 63.4148) -> (331.6692, 82.4848)
  line L146 (319.0992, 82.4848) -> (319.0992, 63.4148)
  line L147 (331.6692, 82.4848) -> (319.0992, 82.4848)
  line L148 (319.0992, 63.4148) -> (331.6692, 63.4148)
  point P0 (254, 0)
  point P1 (254, 0)
  dimension "d76" = 6.35
  dimension "d77" = 12.7
  dimension "d158" = 9.66
  dimension "d159" = 12.57
  dimension "d160" = 19.07
  dimension "d161" = 12.57
  dimension "d162" = 19.07
  constraint vertical L34
  constraint coincident L66.start L98
  constraint collinear L43 L112
  constraint collinear L56 L76
  constraint collinear L76 L85
  constraint collinear L114 L115
  constraint horizontal L25
  constraint vertical L0
  constraint horizontal L7
  constraint coincident L37.start L34
  constraint perpendicular L34 L119
  constraint perpendicular L34 L104
  constraint collinear L34 L37
  constraint collinear L9 L34
  constraint parallel L22 L31
  constraint perpendicular L19 L31
  constraint perpendicular L19 L39
  constraint coincident L28.end L22
  constraint perpendicular L22 L28
  constraint collinear L22 L117
  constraint collinear L111 L117
  constraint horizontal L52
  constraint horizontal L20
  constraint perpendicular L2 L132
  constraint vertical L131
  constraint perpendicular L36 L114
  constraint horizontal L108
  constraint horizontal L45
  constraint horizontal L23
  constraint vertical L74
  constraint vertical L82
  constraint perpendicular L7 L26
  constraint parallel L10 L22
  constraint parallel L14 L111
  constraint vertical L4
  constraint parallel L55 L73
  constraint parallel L66 L136
  constraint parallel L98 L123
  constraint parallel L1 L84
  constraint coincident P1 P0
  constraint parallel L58 L99
  constraint parallel L78 L83
  constraint perpendicular L78 L81
  constraint horizontal L95
  constraint vertical L105
  constraint horizontal L18
  constraint coincident L132.start L18
  constraint coincident L122.end L11
  constraint horizontal L141
  constraint vertical L142
  constraint horizontal L143
  constraint vertical L144
  constraint horizontal L148
  constraint vertical L145
  constraint horizontal L147
  constraint vertical L146
  measures "d76" distance of L19.start L19.end
  measures "d77" distance of L19.end L28.start
  measures "d158" diameter of A0
  measures "d159" distance of L141.start L141.end
  measures "d160" distance of L141.start L143.end
  measures "d161" distance of L146.end L145.start
  measures "d162" distance of L146.end L146.start
extrude "Extrude3" add sketch "Top" along normal blind 6.35 separate body contours L0 L1 L2 L3 L4 L5 L6 L7 L8 L9 L10 L11 L12 L13 L14 L15 L16 L17 L18 L19 L20 L21 L22 L23 L24 L25 L26 L27 L28 L29 L30 L31 L32 L33 L34 L35 L36 L37 L38 L39 L40 L41 L42 L43 L44 L46 L47 L48 L49 L50 L51 L52 L53 L54 L55 L56 L57 L58 L59 L60 L61 L62 L63 L64 L65 L66 L67 L68 L70 L71 L72 L73 L74 L75 L76 L77 L78 L79 L81 L83 L84 L85 L86 L87 L88 L89 L90 L91 L92 L93 L94 L95 L96 L97 L98 L99 L100 L101 L102 L103 L104 L105 L106 L107 L108 L109 L110 L111 L112 L113 L114 L115 L116 L117 L118 L119 L120 L121 L122 L123 L124 L125 L126 L127 L128 L129 L130 L131 L132 L133 L134 L135 L136 L137 L138 L139 L140 makes body 2
copy_body "Body->Comp1" bodies 1 removing the originals makes body 3 in component "Bottom"
copy_body "Body->Comp2" bodies 2 removing the originals makes body 4 in component "Top"
extrude "Extrude4" add sketch "Walls" along normal blind 6.35 separate body makes body 5 at (135.6992, 315.5185, 0) makes body 6 at (276.0765, 407.2301, 0) makes body 7 at (10.7367, 435.3174, 0) makes body 8 at (12.8568, 410.6462, 0) makes body 9 at (115.7527, 438.3751, 0) makes body 10 at (140.9289, 393.2813, 0) makes body 11 at (103.8588, 499.0455, 0) makes body 12 at (80.7761, 621.8581, 0) makes body 13 at (250.154, 485.7454, 0) makes body 14 at (10.6925, 509.8785, 0) makes body 15 at (181.6877, 631.4989, 0) makes body 16 at (277.3925, 509.8785, 0)
copy_body "Body->Comp3" bodies 6 removing the originals makes body 17 in component "Wall1"
copy_body "Body->Comp4" bodies 13 removing the originals makes body 18 in component "Wall2"
copy_body "Body->Comp6" bodies 15 removing the originals makes body 19 in component "Wall4"
copy_body "Body->Comp7" bodies 9 removing the originals makes body 20 in component "Wall5"
copy_body "Body->Comp8" bodies 12 removing the originals makes body 21 in component "Wall6"
copy_body "Body->Comp9" bodies 11 removing the originals makes body 22 in component "Wall7"
copy_body "Body->Comp10" bodies 10 removing the originals makes body 23 in component "Wall8"
copy_body "Body->Comp11" bodies 14 removing the originals makes body 24 in component "Wall9"
copy_body "Body->Comp12" bodies 7 removing the originals makes body 25 in component "Wall10"
copy_body "Body->Comp13" bodies 8 removing the originals makes body 26 in component "Wall11"
copy_body "Body->Comp14" bodies 5 removing the originals makes body 27 in component "Wall12"
move_body "Move1" bodies 21 to x (1, 0, 0) y (0, 1, 0) z (0, 0, 1) at (0, -341.2788, -556.2658) in component "Wall6"
move_body "Move1'" bodies 19 to x (1, 0, 0) y (0, 1, 0) z (0, 0, 1) at (0, -341.2788, -556.2658) in component "Wall4"
move_body "Move1''" bodies 22 to x (1, 0, 0) y (0, 1, 0) z (0, 0, 1) at (0, -341.2788, -556.2658) in component "Wall7"
move_body "Move1'''" bodies 23 to x (1, 0, 0) y (0, 1, 0) z (0, 0, 1) at (0, -341.2788, -556.2658) in component "Wall8"
move_body "Move1''''" bodies 20 to x (1, 0, 0) y (0, 1, 0) z (0, 0, 1) at (0, -341.2788, -556.2658) in component "Wall5"
move_body "Move2" bodies 21 to x (1, 0, 0) y (0, 1, 0) z (0, 0, 1) at (584.2, 0, 558.8) in component "Wall6"
move_body "Move2'" bodies 19 to x (1, 0, 0) y (0, 1, 0) z (0, 0, 1) at (584.2, 0, 558.8) in component "Wall4"
move_body "Move2''" bodies 22 to x (1, 0, 0) y (0, 1, 0) z (0, 0, 1) at (584.2, 0, 558.8) in component "Wall7"
move_body "Move2'''" bodies 23 to x (1, 0, 0) y (0, 1, 0) z (0, 0, 1) at (584.2, 0, 558.8) in component "Wall8"
move_body "Move2''''" bodies 20 to x (1, 0, 0) y (0, 1, 0) z (0, 0, 1) at (584.2, 0, 558.8) in component "Wall5"
copy_body "Body->Comp15" bodies 16 removing the originals makes body 28 in component "Wall3 (1)"